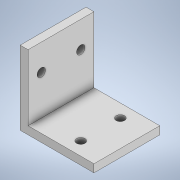
# Autodesk Inventor part: Angle
Saved by Autodesk Inventor 2022 (Build 260153000, 153)
## iProperties
Created: 2023-02-02
Part Number: Angle
Material: Generic
Document SubType Name: Modeling
Designer: Rishi  Agrawal
Density: 1 g/cm^3
Appearance: Default
Author: Rishi  Agrawal
Autodesk Inventor part; units mm, degrees
ref_plane "YZ Plane" through (0, 0, 0) normal (1, 0, 0) x (0, 1, 0)
ref_plane "XZ Plane" through (0, 0, 0) normal (0, 1, 0) x (-1, 0, 0)
ref_plane "XY Plane" through (0, 0, 0) normal (0, 0, 1) x (1, 0, 0)
sketch "Sketch1" plane through (0, 0, 0) normal (1, 0, 0) x (0, 1, 0)
  line L0 (-28, 25) -> (28, 25)
  line L1 (28, 25) -> (28, -25)
  line L2 (28, -25) -> (-28, -25)
  line L3 (-28, -25) -> (-28, 25)
  line L4 (-28, 25) -> (28, -25) construction
  line L5 (28, 25) -> (-28, -25) construction
  point P0 (0, 0)
  dimension "d0" = 56
  dimension "d1" = 50
  constraints: 12 end point, 2 midpoint, 2 parallel, 1 horizontal, 1 perpendicular
  measures "d0" distance of L1.end L2.end
  measures "d1" distance of L0.end L1.end
extrude "Extrusion1" add sketch "Sketch1" along normal blind 6
sketch "Sketch2" plane through (6, 0, 0) normal (1, 0, 0) x (0, 0, -1)
  line L0 (-25, -28) -> (25, -28)
  line L1 (25, -28) -> (25, -22)
  line L2 (25, -22) -> (-25, -22)
  line L3 (-25, -22) -> (-25, -28)
  point P0 (0, 0)
  dimension "d4" = 50
  dimension "d5" = 6
  constraints: 8 end point, 2 parallel, 1 horizontal, 1 perpendicular
  measures "d4" distance of L2.end L1.end
  measures "d5" distance of L1.end L0.end
extrude "Extrusion2" add sketch "Sketch2" along normal blind 50
sketch "Sketch3" plane through (56, -22, 25) normal (0, 1, 0) x (1, 0, 0)
  circle A0 centre (-20, 10) radius 3.2
  circle A1 centre (-20, 40) radius 3.2
  point P0 (-56, 25)
  dimension "d9" = 6.4
  dimension "d10" = 6.4
  constraints: 2 centre point
  measures "d9" diameter of A0
  measures "d10" diameter of A1
sketch "Sketch4" plane through (6, 0, 0) normal (1, 0, 0) x (0, 0, -1)
  circle A0 centre (-15, 8) radius 3.2
  circle A1 centre (15, 8) radius 3.2
  point P0 (0, 0)
  dimension "d11" = 6.4
  dimension "d12" = 6.4
  constraints: 2 centre point
  measures "d11" diameter of A0
  measures "d12" diameter of A1
extrude "Extrusion3" cut sketch "Sketch4" against normal through all
extrude "Extrusion4" cut sketch "Sketch3" against normal through all
body "Solid1"
